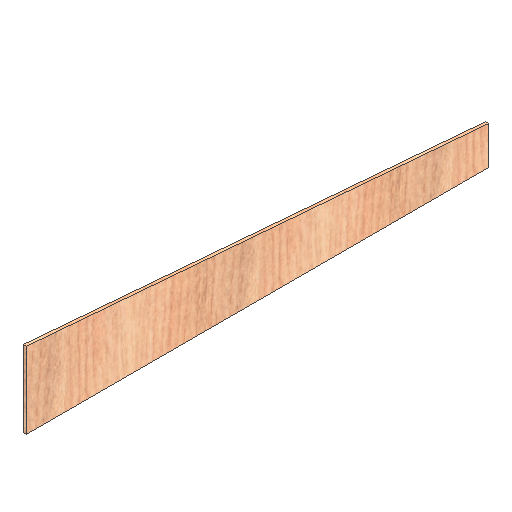
# Autodesk Inventor part: Edge Band - Platform B Flat
Saved by Autodesk Inventor 2021 (Build 250183000, 183)
## iProperties
Created: 2020-05-12
Part Number: Edge Band - Platform B Flat
Material: Wood (Birch)
Document SubType Name: Modeling
Designer: Dan Wikman
Density: 0.55 g/cm^3
Appearance: Birch - Natural Polished
Mass: 99.9702 g
Surface Area: 963.373 cm^2
Volume: 181.764 cm^3
Author: Dan Wikman
Autodesk Inventor part; units mm, degrees
ref_plane "YZ Plane" through (0, 0, 0) normal (1, 0, 0) x (0, 1, 0)
ref_plane "XZ Plane" through (0, 0, 0) normal (0, 1, 0) x (-1, 0, 0)
ref_plane "XY Plane" through (0, 0, 0) normal (0, 0, 1) x (1, 0, 0)
sketch "Sketch1" plane through (0, 0, 0) normal (1, 0, 0) x (0, 1, 0)
  line L0 (62.6437, 415.3628) -> (-37.3563, 415.3628)
  line L1 (-37.3563, 415.3628) -> (-37.3563, -190.5172)
  line L2 (-37.3563, -190.5172) -> (12.6437, -190.5172)
  line L3 (12.6437, -190.5172) -> (62.6437, 415.3628)
  point P0 (0, 0)
  dimension "d4" = 100
  dimension "d6" = 605.88
  dimension "d7" = 50
  constraints: 8 end point, 2 horizontal, 1 perpendicular
  measures "d4" distance of L0.start L0.end
  measures "d6" distance of L0.end L1.end
  measures "d7" distance of L1.end L2.end
extrude "Extrusion1" add sketch "Sketch1" along normal blind 4
body "Solid1"
